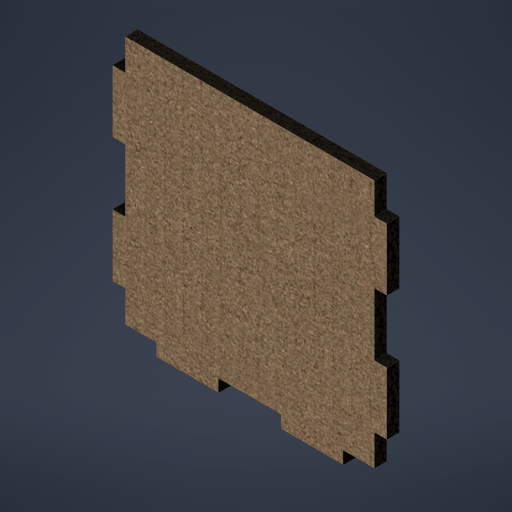
# Autodesk Inventor part: Car_Left
Saved by Autodesk Inventor 2024.1 (Build 281209000, 209)
## iProperties
Created: 2023-08-04
Part Number: Car_Left
Material: MDF Medium Density Fiberboard
Document SubType Name: Modeling
Designer: jaege
Density: 0.8 g/cm^3
Appearance: Cardboard - Corrugated
Author: jaege
Autodesk Inventor part; units mm, degrees
ref_plane "YZ Plane" through (0, 0, 0) normal (1, 0, 0) x (0, 1, 0)
ref_plane "XZ Plane" through (0, 0, 0) normal (0, 1, 0) x (-1, 0, 0)
ref_plane "XY Plane" through (0, 0, 0) normal (0, 0, 1) x (1, 0, 0)
sketch "Sketch1" plane through (0, 0, 0) normal (0, 0, 1) x (1, 0, 0)
  line L0 (0, 0) -> (0, 20) construction
  line L1 (0, 20) -> (-4, 20) projected
  line L2 (-4, 0) -> (-4, 20) projected
  line L3 (0, 0) -> (-4, 0) projected
  line L4 (0, 40) -> (0, 60) construction
  line L5 (0, 60) -> (-4, 60) projected
  line L6 (-4, 40) -> (-4, 60) projected
  line L7 (0, 40) -> (-4, 40) projected
  line L8 (0, 70) -> (-4, 70) construction
  line L9 (0, 70) -> (80, 70)
  line L10 (80, 70) -> (80, 60)
  line L11 (80, -10) -> (0, -10) construction
  line L12 (0, -10) -> (0, 0)
  line L13 (40, 70) -> (40, -10) construction
  line L14 (0, 60) -> (0, 70)
  line L15 (0, 40) -> (0, 60) construction
  line L16 (0, 20) -> (0, 40)
  line L17 (0, 0) -> (0, 20) construction
  line L18 (80, 20) -> (84, 20)
  line L19 (84, 0) -> (84, 20)
  line L20 (80, 0) -> (84, 0)
  line L21 (80, 60) -> (84, 60)
  line L22 (84, 40) -> (84, 60)
  line L23 (80, 40) -> (84, 40)
  line L24 (80, 70) -> (84, 70) construction
  line L25 (80, 60) -> (80, 40) construction
  line L26 (80, 40) -> (80, 20)
  line L27 (80, 20) -> (80, 0) construction
  line L28 (80, 0) -> (80, -10)
  line L29 (10, -10) -> (10, -14)
  line L30 (10, -14) -> (30, -14)
  line L31 (30, -10) -> (30, -14)
  line L32 (50, -10) -> (50, -14)
  line L33 (50, -14) -> (70, -14)
  line L34 (70, -10) -> (70, -14)
  line L35 (10, -10) -> (0, -10)
  line L36 (30, -10) -> (50, -10)
  line L37 (70, -10) -> (80, -10)
  point P0 (40, 30)
  dimension "d0" = 80
  dimension "d1" = 80
  dimension "d6" = 90
  constraints: 70 end point, 26 parallel, 9 symmetric about line, 5 perpendicular, 3 midpoint, 1 horizontal, 15 other
  measures "d0" distance of L11.start L11.end
  measures "d1" distance of L9.end L11.start
extrude "Extrusion1" add sketch "Sketch1" along normal blind 4
body "Solid1"
